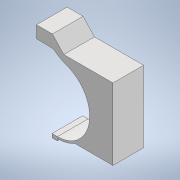
# Autodesk Inventor part: TRIGGER_1
Saved by Autodesk Inventor 2022 (Build 260153000, 153)
## iProperties
Created: 2022-05-17
Part Number: TRIGGER_1
Material: Generic
Document SubType Name: Sheet Metal
Designer: joshn
Density: 1 g/cm^3
Sheet Metal Rule: Default
Appearance: Default
Author: joshn
Autodesk Inventor part; units mm, degrees
ref_plane "YZ Plane" through (0, 0, 0) normal (1, 0, 0) x (0, 1, 0)
ref_plane "XZ Plane" through (0, 0, 0) normal (0, 1, 0) x (-1, 0, 0)
ref_plane "XY Plane" through (0, 0, 0) normal (0, 0, 1) x (1, 0, 0)
sketch "Sketch1" plane through (0, 0, 0) normal (0, 0, 1) x (1, 0, 0)
  line L0 (2.4315, 1.4598) -> (2.4315, 0.2522)
  line L1 (3.9851, -7.1321) -> (3.9851, -7.5057)
  line L2 (10.0394, 0.2522) -> (10.0394, -6.8634)
  line L3 (3.9851, -7.5057) -> (4.5201, -7.4999)
  line L4 (2.4315, 1.4598) -> (4.0193, 1.4598)
  line L5 (4.0193, 1.4598) -> (5.1567, 0.2522)
  line L6 (10.0394, 0.2522) -> (5.1567, 0.2522)
  line L7 (3.8515, 0.2266) -> (2.4315, 0.2522)
  line L8 (3.9851, -7.1321) -> (4.5201, -7.1321)
  line L9 (-0.7118, -7.1321) -> (4.5201, -7.1321) construction
  line L10 (2.5773, -7.521) -> (4.9849, -7.4948) construction
  line L11 (4.5201, -7.4999) -> (4.5201, -7.1321) construction
  line L12 (4.5201, -7.316) -> (4.5622, -7.316)
  arc A0 (4.5622, -7.316) -> (6.2215, -6.8634) centre (4.5622, -4.0479) ccw
  line L13 (6.7434, -6.8634) -> (10.5583, -6.8634) construction
  line L14 (4.5201, -7.4999) -> (4.5201, -7.316)
  line L15 (6.2215, -6.8634) -> (10.0394, -6.8634)
  arc A1 (6.7148, -6.2287) -> (5.4154, -0.5273) centre (4.2722, -3.7866) ccw
  arc A2 (4.3057, 0.0726) -> (5.4154, -0.5273) centre (6.7406, 3.2507) ccw
  arc A3 (4.3057, 0.0726) -> (3.8515, 0.2266) centre (3.8515, -0.5202) ccw
  arc A4 (4.5201, -7.1321) -> (6.7148, -6.2287) centre (4.5341, -4.0485) ccw
  point P0 (0, 0)
extrude "Plate2" add sketch "Sketch1" along normal blind 3.048
equation "\"d1\" = Thickness"
equation "\"BendRadius\" = Thickness"
equation "\"BendReliefWidth\" = Thickness"
equation "\"BendReliefDepth\" = 0.5 * Thickness"
equation "\"CornerReliefSize\" = 4 * Thickness"
equation "\"MinimumRemnant\" = 2 * Thickness"
equation "\"TransitionRadius\" = BendRadius"
equation "\"JacobiRadiusSize\" = BendRadius"
equation "\"GapSize\" = Thickness"
equation "\"Thickness\" = 3.048"
body "Solid2"
